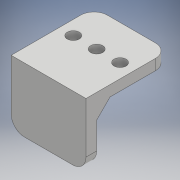
# Autodesk Inventor part: BLTouch
Saved by Autodesk Inventor 2017 (Build 210142000, 142)
## iProperties
Created: 2021-05-05
Part Number: BLTouch
Material: Generic
Document SubType Name: Modeling
Designer: ale
Density: 1 g/cm^3
Appearance: Default
Author: ale
Autodesk Inventor part; units mm, degrees
ref_plane "YZ Plane" through (0, 0, 0) normal (1, 0, 0) x (0, 1, 0)
ref_plane "XZ Plane" through (0, 0, 0) normal (0, 1, 0) x (-1, 0, 0)
ref_plane "XY Plane" through (0, 0, 0) normal (0, 0, 1) x (1, 0, 0)
sketch "Sketch1" plane through (0, 0, 0) normal (0, 0, 1) x (1, 0, 0)
  line L0 (-14, 15.5) -> (14, 15.5)
  line L1 (14, 15.5) -> (14, -15.5)
  line L2 (14, -15.5) -> (-14, -15.5)
  line L3 (-14, -15.5) -> (-14, 15.5)
  line L4 (-14, 15.5) -> (14, -15.5) construction
  line L5 (14, 15.5) -> (-14, -15.5) construction
  point P0 (0, 0)
  dimension "d0" = 28
  dimension "d1" = 31
  constraints: 12 end point, 2 midpoint, 2 parallel, 1 horizontal, 1 perpendicular
  measures "d0" distance of L1.end L2.end
  measures "d1" distance of L0.end L1.end
extrude "Extrusion1" add sketch "Sketch1" along normal blind 4
sketch "Sketch2" plane through (0, 0, 4) normal (0, 0, 1) x (1, 0, 0)
  line L0 (-14, -15.5) -> (14, -15.5) projected
  point P0 (0, 2.5)
  point P1 (-8.75, 2.5)
  point P2 (8.75, 2.5)
  dimension "d7" = 8.75
  dimension "d8" = 8.75
  dimension "d19" = 18
  dimension "d20" = 18
  dimension "d21" = 18
  measures "d7" distance of point (0, 2.5) point (-8.75, 2.5)
  measures "d8" distance of point (8.75, 2.5) point (0, 2.5)
  measures "d19" distance from line of L0 point (8.75, 2.5)
  measures "d20" distance from line of L0 point (0, 2.5)
  measures "d21" distance from line of L0 point (-8.75, 2.5)
hole "Hole1" at (0, 2.5, 4) at (-8.75, 2.5, 4) at (8.75, 2.5, 4) direction (0, 0, -1) diameter 4.5 end through all
sketch "Sketch3" plane through (0, 0, 0) normal (0, 0, -1) x (-1, 0, 0)
  line L0 (14, -15.5) -> (-14, -15.5) projected
  line L1 (14, 15.5) -> (14, -15.5) projected
  line L2 (-14, -15.5) -> (14, -15.5)
  line L3 (14, -15.5) -> (14, -11.5)
  line L4 (14, -11.5) -> (-14, -11.5)
  line L5 (-14, -11.5) -> (-14, -15.5)
  point P0 (0, 0)
  dimension "d16" = 4
  constraints: 8 end point, 2 parallel, 1 horizontal, 1 perpendicular, 1 point on line
  measures "d16" distance of L3.end L2.end
extrude "Extrusion2" add sketch "Sketch3" along normal blind 20
chamfer "Chamfer1" distance 5 angle 45 1 edges at (0, -11.5, 0)
fillet "Fillet1" radius 5 4 edges at (14, 15.5, 2) (-14, 15.5, 2) (14, -13.5, -20) (-14, -13.5, -20)
equation "\"d20\" = d19"
equation "\"d21\" = d19"
body "Solid1"
